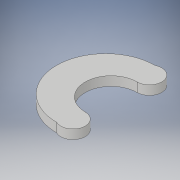
# Autodesk Inventor part: 000.703 - Тяга
Saved by Autodesk Inventor 2019 (Build 230136000, 136)
## iProperties
Created: 2020-02-29
Part Number: 000.703 - Тяга
Material: Типовые
Document SubType Name: Modeling
Designer: Петров Иван
Density: 1 g/cm^3
Appearance: По умолчанию
Author: Петров Иван
Autodesk Inventor part; units mm, degrees
ref_plane "YZ Plane" through (0, 0, 0) normal (1, 0, 0) x (0, 1, 0)
ref_plane "XZ Plane" through (0, 0, 0) normal (0, 1, 0) x (-1, 0, 0)
ref_plane "XY Plane" through (0, 0, 0) normal (0, 0, 1) x (1, 0, 0)
sketch "Эскиз3" plane through (0, 0, 0) normal (0, 1, 0) x (-1, 0, 0)
  arc A0 (1.791, 3.5766) -> (0, -4) centre (0, 0) ccw
  arc A1 (0, -21) -> (1.791, -28.5766) centre (0, -25) ccw
  arc A2 (1.791, -28.5766) -> (1.791, 3.5766) centre (1.791, -12.5) ccw
  arc A3 (0, -21) -> (0, -4) centre (0, -12.5) ccw
  dimension "d12" = 8
  dimension "d13" = 8
  dimension "d14" = 25
  constraints: 12 point on circle, 4 centre point, 1 coincident
  measures "d12" diameter of A0
  measures "d13" diameter of A1
  measures "d14" distance of point (0, 0) A1.centre
extrude "Выдавливание3" add sketch "Эскиз3" along normal blind 3
